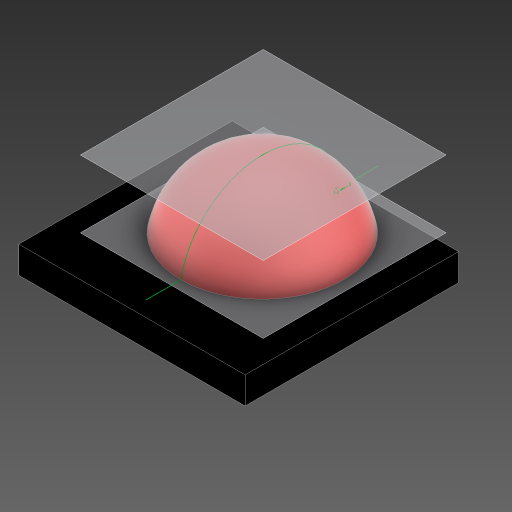
# Autodesk Inventor part: ball_2
Saved by Autodesk Inventor 2023 (Build 270158000, 158)
## iProperties
Created: 2024-09-29
Part Number: ball_2
Material: Типовые
Document SubType Name: Modeling
Designer: Ivan
Density: 1 g/cm^3
Appearance: Шотландка — бежевая
Mass: 212.175 g
Surface Area: 172.034 cm^2
Volume: 212.175 cm^3
Author: Ivan
Autodesk Inventor part; units mm, degrees
ref_plane "YZ Plane" through (0, 0, 0) normal (1, 0, 0) x (0, 1, 0)
ref_plane "XY Plane" through (0, 0, 0) normal (0, 0, 1) x (1, 0, 0)
sketch "Эскиз1" plane through (0, 0, 0) normal (0, 1, 0) x (-1, 0, 0)
  arc A0 (37, 0) -> (-37, 0) centre (0, 0) ccw
  line L0 (37, 0) -> (-37, 0)
  dimension "d0" = 37
  constraints: 2 end point, 2 point on circle, 1 centre point, 1 coincident, 1 horizontal
  measures "d0" radius of A0
revolve "Вращение1" add sketch "Эскиз1" angle 360 about axis through (-37, 0, 0) along (1, 0, 0)
ref_plane "РабПлоскость2" through (0, 7, 0) normal (0, 1, 0) x (-1, 0, 0)
ref_plane "РабПлоскость1" through (0, 37, 0) normal (0, 1, 0) x (-1, 0, 0)
sketch "Эскиз3" plane through (0, 0, 0) normal (1, 0, 0) x (0, 1, 0)
  circle A0 centre (0, 0) radius 37 projected
  line L0 (6.4, -36.4423) -> (6.4, -33.4423)
  line L1 (7.6, -36.211) -> (7.6, -33.4423)
  line L2 (6.4, -33.4423) -> (7.6, -33.4423)
  line L3 (7, 51.8) -> (7, -51.8) projected
  point P0 (7, -33.4423)
  dimension "d3" = 3
  dimension "d4" = 1.2
  constraints: 6 end point, 2 point on circle, 2 vertical, 1 horizontal, 1 midpoint, 1 point on line
  measures "d3" distance of L0.start L0.end
  measures "d4" distance of L0.end L1.end
sketch "Эскиз4" plane through (0, 7, 0) normal (0, 1, 0) x (-1, 0, 0)
  circle A0 centre (0, 0) radius 37.054
  constraints: 1 centre point, 1 coincident
extrude "Выдавливание1" cut sketch "Эскиз4" against normal blind 54.75
sketch "Эскиз5" plane through (0, 7, 0) normal (0, 1, 0) x (-1, 0, 0)
  line L0 (-51.001, -36.3535) -> (49.7571, -36.3535)
  line L1 (49.7571, -36.3535) -> (49.7571, 58.6465)
  line L2 (49.7571, 58.6465) -> (-51.001, 58.6465)
  line L3 (-51.001, 58.6465) -> (-51.001, -36.3535)
  point P0 (0, 0)
  dimension "d9" = 95
  constraints: 8 end point, 2 parallel, 1 horizontal, 1 perpendicular
  measures "d9" distance of L2.end L0.start
extrude "Выдавливание2" add sketch "Эскиз5" against normal blind 12
